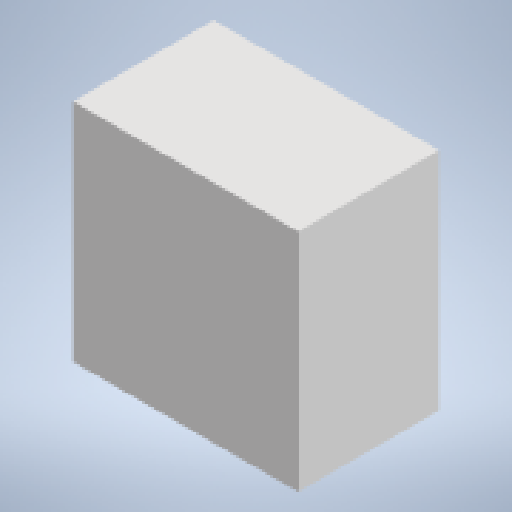
# Autodesk Inventor part: Caja
Saved by Autodesk Inventor 2023 (Build 270158000, 158)
## iProperties
Created: 2023-04-03
Part Number: Caja
Material: Genérico
Document SubType Name: Modeling
Designer: sergi
Density: 1 g/cm^3
Appearance: Valor por defecto
Author: sergi
Autodesk Inventor part; units mm, degrees
ref_plane "YZ Plane" through (0, 0, 0) normal (1, 0, 0) x (0, 1, 0)
ref_plane "XZ Plane" through (0, 0, 0) normal (0, 1, 0) x (-1, 0, 0)
ref_plane "XY Plane" through (0, 0, 0) normal (0, 0, 1) x (1, 0, 0)
sketch "Boceto1" plane through (0, 0, 0) normal (0, 0, 1) x (1, 0, 0)
  circle A0 centre (-35.8, -35.8) radius 2.125 projected
  circle A1 centre (35.8, 35.8) radius 2.125 projected
  circle A2 centre (35.8, -35.8) radius 2.125 projected
  circle A3 centre (-35.8, 35.8) radius 2.125 projected
  line L0 (-40, -40) -> (-40, 40) projected
  line L1 (40, -40) -> (-40, -40) projected
  line L2 (40, 40) -> (40, -40) projected
  line L3 (-40, 40) -> (40, 40) projected
  line L4 (-40, 40) -> (40, 40)
  line L5 (40, 40) -> (40, -40)
  line L6 (40, -40) -> (-40, -40)
  line L7 (-40, -40) -> (-40, 40)
  point P0 (0, 0)
  constraints: 8 end point, 2 parallel, 1 horizontal, 1 perpendicular
extrude "Extrusión1" add sketch "Boceto1" along normal blind 50 contours A0 | A1 | A2 | A3 | L0 L3 L2 L1
sketch "Boceto2" plane through (0, 0, 0) normal (0, 0, -1) x (-1, 0, 0)
  circle A0 centre (35.8, 35.8) radius 2.125 projected
  circle A1 centre (35.8, -35.8) radius 2.125 projected
  circle A2 centre (-35.8, -35.8) radius 2.125 projected
  circle A3 centre (-35.8, 35.8) radius 2.125 projected
  point P0 (0, 0)
hole "Agujero1" at (-35.8, 35.8, 0) at (-35.8, -35.8, 0) at (35.8, -35.8, 0) at (35.8, 35.8, 0) direction (0, 0, 1) diameter 4.25 depth 10
shell "Vaciado1" thickness 2.2 removed faces 1 at (11.4636, -11.4031, 0)
sketch "Boceto3" plane through (37.8, 37.8, 47.8) normal (0, 0, -1) x (-1, 0, 0)
  circle A0 centre (65.17, -21.6591) radius 1.4999 projected
  circle A1 centre (61.425, -71.3162) radius 1.5 projected
  line L0 (75.6, 0) -> (75.6, -75.6) projected
  line L1 (0, 0) -> (75.6, 0) projected
  line L2 (0, -75.6) -> (0, 0) projected
  line L3 (75.6, -75.6) -> (0, -75.6) projected
  circle A2 centre (7.2236, -56.9604) radius 1.5 projected
  circle A3 centre (6.6748, -24.2806) radius 1.5001 projected
  circle A4 centre (65.17, -21.6591) radius 3
  circle A5 centre (61.425, -71.3162) radius 3
  circle A6 centre (7.2236, -56.9604) radius 3
  circle A7 centre (6.6748, -24.2806) radius 3
  point P0 (37.8, -37.8)
  dimension "d10" = 6
  dimension "d11" = 6
  dimension "d12" = 6
  dimension "d13" = 6
  constraints: 4 centre point, 4 coincident
  measures "d10" diameter of A4
  measures "d11" diameter of A5
  measures "d12" diameter of A6
  measures "d13" diameter of A7
extrude "Extrusión2" add sketch "Boceto3" along normal blind 5 contours A4 | A5 | A6 | A7
fillet "Empalme1" radius 2 4 edges at (-20.625, -33.5162, 47.8) (33.5764, -19.1604, 47.8) (34.1252, 13.5194, 47.8) (-24.37, 16.1409, 47.8)
sketch "Boceto4" plane through (-37.8, -37.8, 47.8) normal (1, 0, 0) x (0, 0, -1)
  line L0 (14.2955, 12.3019) -> (14.2955, 19.7876) projected
  line L1 (14.2955, 19.7876) -> (7, 19.9181) projected
  line L2 (7, 12.3019) -> (14.2955, 12.3019) projected
  line L3 (14.2955, 12.3019) -> (7, 12.3019)
  line L4 (7, 12.3019) -> (7, 19.9181)
  line L5 (7, 19.9181) -> (14.2955, 19.9181)
  line L6 (14.2955, 19.9181) -> (14.2955, 12.3019)
  line L7 (6, 20.9181) -> (6, 11.3019)
  line L8 (6, 11.3019) -> (15.2955, 11.3019)
  line L9 (15.2955, 11.3019) -> (15.2955, 20.9181)
  line L10 (15.2955, 20.9181) -> (6, 20.9181)
  point P0 (47.8, 37.8)
  dimension "d17" = 1
  constraints: 16 end point, 4 parallel, 2 perpendicular, 1 horizontal, 3 other
  measures "d17" distance between parallel lines of L4 L7
extrude "Extrusión3" cut sketch "Boceto4" against normal blind 5 contours L2 L4 L1 L0 | L1 L5 L6 | L10 L9 L8 L7
